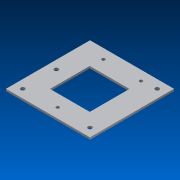
# Autodesk Inventor part: Window_MotorMounting
Saved by Autodesk Inventor 2013 (Build 170138000, 138)
## iProperties
Created: 2013-07-16
Part Number: Window_MotorMounting
Material: Aluminum 6061
Document SubType Name: Modeling
Designer: orange
Density: 1 g/cm^3
Author: orange
Autodesk Inventor part; units mm, degrees
ref_plane "YZ Plane" through (0, 0, 0) normal (1, 0, 0) x (0, 1, 0)
ref_plane "XZ Plane" through (0, 0, 0) normal (0, 1, 0) x (-1, 0, 0)
ref_plane "XY Plane" through (0, 0, 0) normal (0, 0, 1) x (1, 0, 0)
sketch "Sketch2" plane through (0, 0, 0) normal (0, 1, 0) x (-1, 0, 0)
  line L0 (0, 0) -> (-101.6, 0)
  line L1 (-101.6, 0) -> (-101.6, -127)
  line L2 (-101.6, -127) -> (0, -127)
  line L3 (0, -127) -> (0, 0)
  dimension "d0" = 127
  dimension "d1" = 101.6
  constraints: 8 end point, 2 parallel, 1 horizontal, 1 perpendicular
  measures "d0" distance of L2.end L0.start
  measures "d1" distance of L0.start L0.end
extrude "Extrusion1" add sketch "Sketch2" along normal blind 3.175
sketch "Sketch3" plane through (0, 3.175, 0) normal (0, 1, 0) x (1, 0, 0)
  line L0 (101.6, 127) -> (0, 127) projected
  line L1 (35.12, 112.2299) -> (63.5, 14.7782)
  line L2 (63.5, 14.7782) -> (91.88, 112.2299)
  line L3 (0, 127) -> (0, 0) projected
  line L4 (0, 0) -> (101.6, 0) projected
  dimension "d5" = 14.7701
  dimension "d6" = 14.7701
  dimension "d9" = 56.76
  dimension "d27" = 101.5
  dimension "d28" = 101.5
  dimension "d58" = 63.5
  dimension "d60" = 97.4517
  dimension "d61" = 14.7782
  constraints: 4 end point, 1 coincident
  measures "d5" distance from line of L2.end L0
  measures "d6" distance from line of L1.start L0
  measures "d9" distance of L1.start L2.end
  measures "d27" distance of L1.end L2.end
  measures "d28" distance of L1.start L1.end
  measures "d58" distance from line of L3 point (63.5, 14.778)
  measures "d60" vertical distance of L1.end L2.end
  measures "d61" distance from line of L4 L1.end
hole "Hole1" at (35.12, 3.175, -112.2299) at (91.88, 3.175, -112.2299) at (63.5, 3.175, -14.7782) direction (0, -1, 0) diameter 5 end through all
sketch "Sketch5" plane through (0, 0, 0) normal (0, -1, 0) x (1, 0, 0)
  circle A0 centre (91.88, -112.2299) radius 2.5 projected
  circle A1 centre (35.12, -112.2299) radius 2.5 projected
  line L0 (63.5, -63.1355) -> (91.88, -112.2299)
  line L1 (33.5, -93.1355) -> (93.5, -93.1355)
  line L2 (93.5, -93.1355) -> (93.5, -33.1355)
  line L3 (93.5, -33.1355) -> (33.5, -33.1355)
  line L4 (33.5, -33.1355) -> (33.5, -93.1355)
  line L5 (33.5, -93.1355) -> (93.5, -33.1355) construction
  line L6 (93.5, -93.1355) -> (33.5, -33.1355) construction
  dimension "d33" = 56.707
  dimension "d34" = 56.707
  dimension "d56" = 60
  dimension "d57" = 60
  constraints: 14 end point, 2 midpoint, 2 parallel, 1 horizontal, 1 perpendicular
  measures "d33" distance of A1.centre L0.start
  measures "d34" distance of L0.start L0.end
  measures "d56" distance between parallel lines of L4 L2
  measures "d57" distance of L3.end L1.start
extrude "Extrusion2" cut sketch "Sketch5" against normal blind 25.4 contours L1 L4 L3 L2
sketch "Sketch6" plane through (101.6, 0, 0) normal (1, 0, 0) x (0, 0, -1)
  line L0 (0, 0) -> (127, 0) projected
  line L1 (127, 0) -> (127, 3.175) projected
  line L2 (0, 0) -> (127, 0)
  line L3 (127, 0) -> (127, 3.175)
  line L4 (127, 3.175) -> (0, 3.175)
  line L5 (0, 3.175) -> (0, 0)
  constraints: 8 end point, 2 parallel, 1 horizontal, 1 perpendicular
extrude "Extrusion3" add sketch "Sketch6" along normal blind 25.4
sketch "Sketch7" plane through (0, 3.175, 0) normal (0, 1, 0) x (1, 0, 0)
  line L0 (0, 0) -> (127, 0) projected
  line L1 (127, 127) -> (127, 0) projected
  line L2 (0, 127) -> (127, 127) projected
  line L3 (0, 127) -> (0, 0) projected
  point P0 (12.7, 63.5)
  point P1 (114.3, 114.3)
  point P2 (114.3, 12.7)
  point P3 (12.7, 12.7)
  dimension "d39" = 63.5
  dimension "d40" = 12.7
  dimension "d41" = 12.7
  dimension "d42" = 12.7
  dimension "d43" = 12.7
  dimension "d44" = 12.7
  dimension "d45" = 12.7
  dimension "d46" = 113.5923
  dimension "d47" = 101.6
  dimension "d48" = 50.8
  dimension "d59" = 101.6
  measures "d39" distance from line of point (12.7, 63.5) L2
  measures "d40" distance from line of L3 point (12.7, 63.5)
  measures "d41" distance from line of point (114.3, 114.3) L1
  measures "d42" distance from line of point (114.3, 114.3) L2
  measures "d43" distance from line of L0 point (114.3, 12.7)
  measures "d44" distance from line of L0 point (12.7, 12.7)
  measures "d45" distance from line of point (12.7, 12.7) L3
  measures "d46" distance of point (114.3, 114.3) point (12.7, 63.5)
  measures "d47" distance of point (12.7, 12.7) point (114.3, 12.7)
  measures "d48" distance of point (12.7, 12.7) point (12.7, 63.5)
  measures "d59" distance of point (114.3, 12.7) point (114.3, 114.3)
hole "Hole2" at (12.7, 3.175, -63.5) at (114.3, 3.175, -114.3) at (114.3, 3.175, -12.7) at (12.7, 3.175, -12.7) direction (0, -1, 0) diameter 6.35 end through all
body "Solid1"
